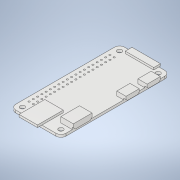
# Autodesk Inventor part: pizero_model no gpio
Saved by Autodesk Inventor 2020 (Build 240168000, 168)
## iProperties
Created: 2019-08-11
Part Number: pizero_model no gpio
Material: UHMW, Black
Document SubType Name: Modeling
Designer: mulve
Density: 0.94 g/cm^3
Appearance: White
Author: mulve
Autodesk Inventor part; units mm, degrees
ref_plane "YZ Plane" through (0, 0, 0) normal (1, 0, 0) x (0, 1, 0)
ref_plane "XZ Plane" through (0, 0, 0) normal (0, 1, 0) x (-1, 0, 0)
ref_plane "XY Plane" through (0, 0, 0) normal (0, 0, 1) x (1, 0, 0)
sketch "Sketch1" plane through (0, 0, 0) normal (0, 1, 0) x (-1, 0, 0)
  line L0 (0, 0) -> (30, 0)
  line L1 (30, 0) -> (30, -65)
  line L2 (30, -65) -> (0, -65)
  line L3 (0, -65) -> (0, 0)
  circle A0 centre (26.5, -3.5) radius 1.375
  circle A1 centre (3.5, -3.5) radius 1.375
  circle A2 centre (26.5, -61.5) radius 1.375
  circle A3 centre (3.5, -61.5) radius 1.375
  line L4 (15, 0) -> (15, -65)
  line L5 (30, -32.5) -> (0, -32.5)
  dimension "d0" = 65
  dimension "d1" = 30
  dimension "d2" = 3.5
  dimension "d3" = 3.5
  dimension "d4" = 3.5
  dimension "d5" = 3.5
  dimension "d6" = 3.5
  dimension "d7" = 3.5
  dimension "d8" = 3.5
  dimension "d9" = 3.5
  dimension "d10" = 2.75
  dimension "d11" = 2.75
  dimension "d12" = 2.75
  dimension "d13" = 2.75
  dimension "d14" = 15
  dimension "d15" = 32.5
  constraints: 12 end point, 4 centre point, 4 coincident, 4 midpoint, 3 perpendicular, 2 parallel, 1 horizontal
  measures "d0" distance of L0.end L1.end
  measures "d1" distance of L1.end L2.end
  measures "d2" distance from line of L1 point (26.5, -3.5)
  measures "d3" distance from line of L0 point (26.5, -3.5)
  measures "d4" distance from line of L0 point (3.5, -3.5)
  measures "d5" distance from line of L3 point (3.5, -3.5)
  measures "d6" distance from line of L3 point (3.5, -61.5)
  measures "d7" distance from line of L2 point (3.5, -61.5)
  measures "d8" distance from line of L2 point (26.5, -61.5)
  measures "d9" distance from line of L1 point (26.5, -61.5)
  measures "d10" diameter of A0
  measures "d11" diameter of A1
  measures "d12" diameter of A2
  measures "d13" diameter of A3
  measures "d14" distance between parallel lines of L1 L4
  measures "d15" distance between parallel lines of L0 L5
extrude "Extrusion1" add sketch "Sketch1" along normal blind 1.5
fillet "Fillet1" radius 3 4 edges at (-30, 0.75, 0) (0, 0.75, 0) (0, 0.75, -65) (-30, 0.75, -65)
sketch "Sketch2" plane through (0, 1.5, 0) normal (0, 1, 0) x (1, 0, 0)
  line L0 (-6.9, 6.8) -> (0.6, 6.8)
  line L1 (0.6, 6.8) -> (0.6, 18)
  line L2 (0.6, 18) -> (-6.9, 18)
  line L3 (-6.9, 18) -> (-6.9, 6.8)
  line L4 (-27, 0) -> (-3, 0) projected
  line L5 (-15, 0) -> (-15, 64.9233)
  line L6 (-30, 62) -> (-30, 3) projected
  line L7 (0.6, 12.4) -> (-6.9, 12.4)
  line L8 (-4.1, 57.95) -> (1.4, 57.95)
  line L9 (1.4, 57.95) -> (1.4, 50.05)
  line L10 (1.4, 50.05) -> (-4.1, 50.05)
  line L11 (-4.1, 50.05) -> (-4.1, 57.95)
  line L12 (-4.1, 45.35) -> (1.4, 45.35)
  line L13 (1.4, 45.35) -> (1.4, 37.45)
  line L14 (1.4, 37.45) -> (-4.1, 37.45)
  line L15 (-4.1, 37.45) -> (-4.1, 45.35)
  line L16 (-4.1, 41.4) -> (1.4, 41.4)
  line L17 (-4.1, 54) -> (1.4, 54)
  line L18 (-22.4, 12.8) -> (-11.4, 12.8)
  line L19 (-11.4, 12.8) -> (-11.4, -2.6)
  line L20 (-11.4, -2.6) -> (-22.4, -2.6)
  line L21 (-22.4, -2.6) -> (-22.4, 12.8)
  line L22 (-16.9, 12.8) -> (-16.9, -2.6)
  line L23 (0, 3) -> (0, 62) projected
  line L24 (-23.5, 65.9) -> (-6.5, 65.9)
  line L25 (-6.5, 65.9) -> (-6.5, 61.9)
  line L26 (-6.5, 61.9) -> (-23.5, 61.9)
  line L27 (-23.5, 61.9) -> (-23.5, 65.9)
  line L28 (-15, 65.9) -> (-15, 61.9)
  point P0 (0, 0)
  dimension "d19" = 11.2
  dimension "d20" = 7.5
  dimension "d21" = 15
  dimension "d23" = 12.4
  dimension "d24" = 7.9
  dimension "d25" = 7.9
  dimension "d26" = 5.5
  dimension "d27" = 3.95
  dimension "d28" = 3.95
  dimension "d29" = 41.4
  dimension "d30" = 54
  dimension "d32" = 30.6
  dimension "d33" = 31.4
  dimension "d34" = 11
  dimension "d35" = 15.4
  dimension "d36" = 2.6
  dimension "d37" = 5.5
  dimension "d38" = 16.9
  dimension "d39" = 65.9
  dimension "d40" = 4
  dimension "d41" = 17
  dimension "d42" = 8.5
  dimension "d43" = 15
  constraints: 52 end point, 11 midpoint, 10 parallel, 7 perpendicular, 6 horizontal, 2 point on line, 1 vertical
  measures "d19" distance of L0.end L1.end
  measures "d20" distance of L1.end L2.end
  measures "d21" distance between parallel lines of L6 L5
  measures "d23" distance between parallel lines of L4 L7
  measures "d24" distance of L8.end L9.end
  measures "d25" distance of L12.end L13.end
  measures "d26" distance of L8.start L8.end
  measures "d27" distance between parallel lines of L14 L16
  measures "d28" distance between parallel lines of L10 L17
  measures "d29" distance between parallel lines of L4 L16
  measures "d30" distance between parallel lines of L4 L17
  measures "d32" distance between parallel lines of L6 L1
  measures "d33" distance between parallel lines of L6 L13
  measures "d34" distance of L19.end L20.end
  measures "d35" distance of L18.end L19.end
  measures "d36" distance between parallel lines of L4 L20
  measures "d37" distance between parallel lines of L21 L22
  measures "d38" distance between parallel lines of L23 L22
  measures "d39" distance between parallel lines of L4 L24
  measures "d40" distance of L26.end L24.start
  measures "d41" distance of L25.end L26.end
  measures "d42" distance between parallel lines of L28 L27
  measures "d43" distance between parallel lines of L6 L28
extrude "Extrusion2" add sketch "Sketch2" along normal blind 3.25 contours L3 L7 L23 L0 | L23 L7 L1 L0 | L3 L2 L23 L7 | L23 L2 L1 L7
extrude "Extrusion3" add sketch "Sketch2" along normal blind 2.55 contours L10 L11 L17 L23 | L23 L17 L9 L10 | L14 L15 L16 L23 | L23 L16 L13 L14 | L23 L12 L13 L16 | L16 L15 L12 L23 | L23 L8 L9 L17 | L17 L11 L8 L23
extrude "Extrusion4" add sketch "Sketch2" along normal blind 1.25 contours L26 L27 L24 L28 L5 | L5 L28 L24 L25 L26
extrude "Extrusion5" add sketch "Sketch2" along normal blind 1.35 contours L21 L18 L22 L4 | L4 L22 L20 L21 | L22 L18 L5 L4 | L4 L19 L20 L22 | L5 L18 L19 L4
chamfer "Chamfer1" distance 1.1735 angle 45 2 edges at (0.3, 1.5, -6.8) (0.3, 1.5, -18)
chamfer "Chamfer2" distance 0.889 angle 45 4 edges at (0.7, 1.5, -37.45) (0.7, 1.5, -45.35) (0.7, 1.5, -50.05) (0.7, 1.5, -57.95)
sketch "Sketch4" plane through (0, 1.5, 0) normal (0, 1, 0) x (1, 0, 0)
  line L0 (-28.85, 7.05) -> (-23.35, 7.05) construction
  line L1 (-23.35, 7.05) -> (-23.35, 57.95) construction
  line L2 (-23.35, 57.95) -> (-28.85, 57.95) construction
  line L3 (-28.85, 57.95) -> (-28.85, 7.05) construction
  line L4 (-30, 62) -> (-30, 3) construction
  line L5 (-27, 0) -> (-22.4, 0) construction
  line L6 (-23.5, 65) -> (-27, 65) construction
  line L7 (-27.37, 8.37) -> (-28.85, 8.37) construction
  line L8 (-24.83, 8.37) -> (-23.35, 8.37) construction
  line L9 (-27.37, 8.37) -> (-27.37, 7.05) construction
  line L10 (-27.37, 56.63) -> (-27.37, 57.95) construction
  line L11 (-24.83, 8.37) -> (-24.83, 7.05) construction
  line L12 (-24.83, 56.63) -> (-24.83, 57.95) construction
  circle A0 centre (-27.37, 8.37) radius 0.508
  circle A1 centre (-27.37, 10.91) radius 0.508
  circle A2 centre (-27.37, 13.45) radius 0.508
  circle A3 centre (-27.37, 15.99) radius 0.508
  circle A4 centre (-27.37, 18.53) radius 0.508
  circle A5 centre (-27.37, 21.07) radius 0.508
  circle A6 centre (-27.37, 23.61) radius 0.508
  circle A7 centre (-27.37, 26.15) radius 0.508
  circle A8 centre (-27.37, 28.69) radius 0.508
  circle A9 centre (-27.37, 31.23) radius 0.508
  circle A10 centre (-27.37, 33.77) radius 0.508
  circle A11 centre (-27.37, 36.31) radius 0.508
  circle A12 centre (-27.37, 38.85) radius 0.508
  circle A13 centre (-27.37, 41.39) radius 0.508
  circle A14 centre (-27.37, 43.93) radius 0.508
  circle A15 centre (-27.37, 46.47) radius 0.508
  circle A16 centre (-27.37, 49.01) radius 0.508
  circle A17 centre (-27.37, 51.55) radius 0.508
  circle A18 centre (-27.37, 54.09) radius 0.508
  circle A19 centre (-27.37, 56.63) radius 0.508
  circle A20 centre (-24.83, 8.37) radius 0.508
  circle A21 centre (-24.83, 10.91) radius 0.508
  circle A22 centre (-24.83, 13.45) radius 0.508
  circle A23 centre (-24.83, 15.99) radius 0.508
  circle A24 centre (-24.83, 18.53) radius 0.508
  circle A25 centre (-24.83, 21.07) radius 0.508
  circle A26 centre (-24.83, 23.61) radius 0.508
  circle A27 centre (-24.83, 26.15) radius 0.508
  circle A28 centre (-24.83, 28.69) radius 0.508
  circle A29 centre (-24.83, 31.23) radius 0.508
  circle A30 centre (-24.83, 33.77) radius 0.508
  circle A31 centre (-24.83, 36.31) radius 0.508
  circle A32 centre (-24.83, 38.85) radius 0.508
  circle A33 centre (-24.83, 41.39) radius 0.508
  circle A34 centre (-24.83, 43.93) radius 0.508
  circle A35 centre (-24.83, 46.47) radius 0.508
  circle A36 centre (-24.83, 49.01) radius 0.508
  circle A37 centre (-24.83, 51.55) radius 0.508
  circle A38 centre (-24.83, 54.09) radius 0.508
  circle A39 centre (-24.83, 56.63) radius 0.508
  point P0 (0, 0)
  point P1 (-27.37, 21.07)
  point P2 (-27.37, 26.15)
  point P3 (-27.37, 31.23)
  point P4 (-27.37, 36.31)
  point P5 (-27.37, 51.55)
  point P6 (-24.83, 21.07)
  point P7 (-24.83, 26.15)
  point P8 (-24.83, 31.23)
  point P9 (-24.83, 36.31)
  point P10 (-24.83, 51.55)
  dimension "d63" = 1.15
  dimension "d64" = 50.9
  dimension "d65" = 7.05
  dimension "d66" = 7.05
  dimension "d67" = 5.5
  dimension "d68" = 2.54
  dimension "d71" = 2.54
  dimension "d74" = 2.54
  dimension "d77" = 1.016
  dimension "d80" = 2.54
  dimension "d83" = 2.54
  constraints: 40 centre point, 20 end point, 9 point on line, 4 perpendicular, 3 collinear, 3 horizontal, 2 parallel, 2 vertical, 117 other
  measures "d63" distance between parallel lines of L4 L3
  measures "d64" distance of L2.end L0.start
  measures "d65" distance between parallel lines of L5 L0
  measures "d66" distance between parallel lines of L6 L2
  measures "d67" distance of L1.end L2.end
  measures "d68" distance of L8.start L7.start
  measures "d71" distance of L7.start point (-27.37, 10.91)
  measures "d74" distance of L7.start point (-24.83, 8.37)
  measures "d77" diameter of A0
  measures "d80" distance of A0.centre A1.centre
  measures "d83" distance of A0.centre A20.centre
extrude "Extrusion7" cut sketch "Sketch4" against normal through all
equation "\"d3\" = d2"
equation "\"d4\" = d3"
equation "\"d5\" = d2"
equation "\"d6\" = d2"
equation "\"d7\" = d3"
equation "\"d8\" = d3"
equation "\"d9\" = d2"
equation "\"d11\" = d10"
equation "\"d12\" = d10"
equation "\"d13\" = d10"
equation "\"d14\" = 0.5 * d1"
equation "\"d15\" = 0.5 * d0"
equation "\"d21\" = d14"
equation "\"d25\" = d24"
equation "\"d27\" = 0.5 * d25"
equation "\"d37\" = 0.5 * d34"
equation "\"d42\" = 0.5 * d41"
equation "\"d43\" = d14"
equation "\"d65\" = d66"
body "Solid1"
